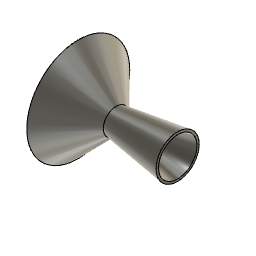
v1 (Autodesk Fusion 360 design; units mm, degrees)
Autodesk Fusion 360 part; units mm, degrees
sketch "Sketch1" plane through (0, 0, 0) normal (0, 0, 1) x (1, 0, 0)
  line L0 (-256.6723, -0.4736) -> (-256.6723, 329.5264)
  line L1 (-256.6723, 329.5264) -> (0, 68.5)
  line L2 (419.4936, -0.4736) -> (419.4936, 130.3264)
  arc A0 (0, 68.5) -> (419.4936, 130.3264) centre (0, 1522.5504) ccw
  line L3 (419.4936, -0.4736) -> (-256.6723, -0.4736)
  line L4 (-256.6723, 348.9802) -> (0.9034, 87.0351)
  line L5 (0.9034, 87.0351) -> (418.3857, 145.844)
  line L6 (418.3857, 145.844) -> (419.4936, 130.3264)
  line L7 (-256.6723, 348.9802) -> (-256.6723, 329.5264)
  dimension "d1" = 68.5
  dimension "d3" = 330
  dimension "d5" = 130.8
  constraint vertical L0
  constraint vertical L2
  constraint perpendicular L2 L3
  constraint parallel L1 L4
  constraint parallel L0 L7
  measures "d1" distance of origin L1.end
  measures "d3" distance of L0.start L0.end
  measures "d5" distance of L2.start L2.end
revolve "Revolve1" add sketch "Sketch1" angle 360 about axis through (419.4936, -0.4736, 0) along (-1, 0, 0) contours L1 A0 L4 L5 L6 L7
